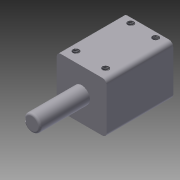
# Autodesk Inventor part: p60 gearbox proxy
Saved by Autodesk Inventor 2011 SP1 (Build 150282100, 282)
## iProperties
Created: 2012-01-19
Part Number: p60 gearbox proxy
Document SubType Name: Modeling
Designer: Christopher
Density: 1 g/cm^3
Author: Christopher
Autodesk Inventor part; units mm, degrees
ref_plane "YZ Plane" through (0, 0, 0) normal (1, 0, 0) x (0, 1, 0)
ref_plane "XZ Plane" through (0, 0, 0) normal (0, 1, 0) x (-1, 0, 0)
ref_plane "XY Plane" through (0, 0, 0) normal (0, 0, 1) x (1, 0, 0)
sketch "Sketch1" plane through (0, 0, 0) normal (0, 0, 1) x (1, 0, 0)
  line L0 (-10.0849, -28.7582) -> (28.0151, -28.7582)
  line L1 (28.0151, -28.7582) -> (28.0151, 9.3418)
  line L2 (28.0151, 9.3418) -> (-10.0849, 9.3418)
  line L3 (-10.0849, 9.3418) -> (-10.0849, -28.7582)
  circle A0 centre (8.9651, -9.7082) radius 6.35
  point P0 (0, 0)
  point P1 (8.9651, 9.3418)
  point P2 (-10.0849, -9.7082)
  dimension "d0" = 38.1
  dimension "d1" = 38.1
  dimension "d4" = 12.7
  constraints: 8 end point, 2 midpoint, 2 parallel, 1 centre point, 1 coincident, 1 horizontal, 1 horizontal alignment, 1 perpendicular, 1 vertical alignment
  measures "d0" distance of L1.end L2.end
  measures "d1" distance of L2.end L0.start
  measures "d4" diameter of A0
extrude "Extrusion1" add sketch "Sketch1" against normal blind 50.8 contours L3 L2 L1 L0 | A0
extrude "Extrusion2" add sketch "Sketch1" along normal blind 38.1 contours A0
fillet "Fillet1" radius 1.5875 1 edges at (2.6151, -9.7082, 38.1)
fillet "Fillet2" radius 3.175 4 edges at (28.0151, 9.3418, -25.4) (-10.0849, 9.3418, -25.4) (28.0151, -28.7582, -25.4) (-10.0849, -28.7582, -25.4)
sketch "Sketch2" plane through (8.9651, -9.7082, 38.1) normal (0, 0, 1) x (1, 0, 0)
  circle A0 centre (0, 0) radius 4.7625 projected
  line L0 (-4.7625, -1.5875) -> (-4.7625, 1.5875)
  line L1 (-4.7625, 1.5875) -> (-7.9375, 1.5875)
  line L2 (-7.9375, 1.5875) -> (-7.9375, -1.5875)
  line L3 (-7.9375, -1.5875) -> (-4.7625, -1.5875)
  point P0 (-8.9651, 9.7082)
  dimension "d13" = 3.175
  dimension "d14" = 1.5875
  dimension "d15" = 3.175
  constraints: 8 end point, 2 perpendicular, 1 parallel, 1 vertical
  measures "d13" distance of L0.start L0.end
  measures "d14" vertical distance of A0.centre L0.start
  measures "d15" distance of L0.end L1.end
extrude "Extrusion3" cut sketch "Sketch2" against normal blind 25.4 contours L0 L3 L2 L1
sketch "Sketch3" plane through (-6.9099, 9.3418, 0) normal (0, 1, 0) x (1, 0, 0)
  line L0 (31.75, 0) -> (0, 0) projected
  line L1 (31.75, 50.8) -> (0, 50.8) projected
  line L2 (-3.175, 50.8) -> (-3.175, 0) projected
  point P0 (6.9099, 0)
  point P1 (26.5665, 7.62)
  point P2 (25.4, 46.99)
  point P3 (6.35, 46.99)
  point P4 (3.8887, 7.62)
  point P5 (34.925, 50.8)
  dimension "d18" = 7.62
  dimension "d19" = 7.62
  dimension "d20" = 3.81
  dimension "d21" = 3.81
  dimension "d22" = 9.525
  dimension "d23" = 9.525
  measures "d18" distance from line of L0 point (26.566, 7.62)
  measures "d19" distance from line of L0 point (3.889, 7.62)
  measures "d20" distance from line of L1 point (25.4, 46.99)
  measures "d21" distance from line of L1 point (6.35, 46.99)
  measures "d22" distance from line of L2 point (6.35, 46.99)
  measures "d23" horizontal distance of point (34.925, 50.8) point (25.4, 46.99)
hole "Hole1" at (19.6566, 9.3418, -7.62) at (18.4901, 9.3418, -46.99) at (-0.5599, 9.3418, -46.99) at (-3.0212, 9.3418, -7.62) direction (0, -1, 0) diameter 4.826 depth 7.62 tip angle 118
thread "Thread1" size "10-32 UNF" class "2B" standard "ANSI Unified Screw Threads" full length
thread "Thread2" size "10-24 UNC" class "2B" standard "ANSI Unified Screw Threads" full length
thread "Thread3" size "10-24 UNC" class "2B" standard "ANSI Unified Screw Threads" full length
thread "Thread4" size "10-24 UNC" class "2B" standard "ANSI Unified Screw Threads" full length
sketch "Sketch4" plane through (0, 0, -50.8) normal (0, 0, -1) x (-1, 0, 0)
  point P0 (0, 0)
  point P1 (-8.9651, -9.7082)
hole "Hole2" at (8.9651, -9.7082, -50.8) direction (0, 0, 1) diameter 5.08 depth 7.62 tip angle 118
body "Solid1"
